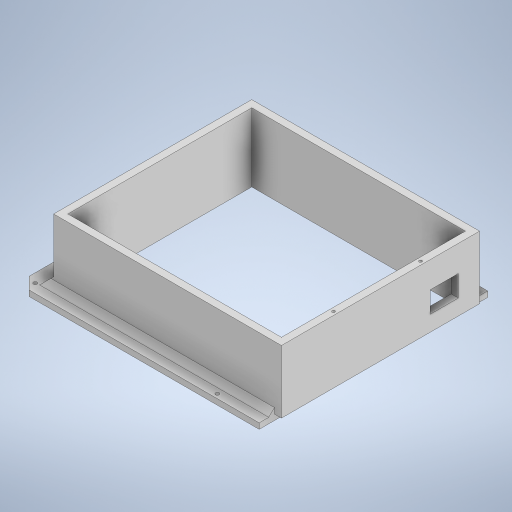
# Autodesk Inventor part: battery holder
Saved by Autodesk Inventor 2023 (Build 270158000, 158)
## iProperties
Created: 2023-08-22
Part Number: battery holder
Material: Generic
Document SubType Name: Modeling
Designer: alian
Density: 1 g/cm^3
Appearance: Default
Author: alian
Autodesk Inventor part; units mm, degrees
ref_plane "YZ Plane" through (0, 0, 0) normal (1, 0, 0) x (0, 1, 0)
ref_plane "XZ Plane" through (0, 0, 0) normal (0, 1, 0) x (-1, 0, 0)
ref_plane "XY Plane" through (0, 0, 0) normal (0, 0, 1) x (1, 0, 0)
sketch "Sketch1" plane through (0, 0, 0) normal (0, 1, 0) x (-1, 0, 0)
  line L0 (0, 0) -> (161, 0)
  line L1 (161, 0) -> (161, -140)
  line L2 (161, -140) -> (0, -140)
  line L3 (0, -140) -> (0, 0)
  line L4 (156, -135) -> (156, -5)
  line L5 (156, -5) -> (5, -5)
  line L6 (5, -5) -> (5, -135)
  line L7 (5, -135) -> (156, -135)
  dimension "d28" = 151
  dimension "d29" = 130
  dimension "d30" = 5
  constraints: 16 end point, 4 parallel, 2 perpendicular, 1 horizontal, 3 other
  measures "d28" distance between parallel lines of L6 L4
  measures "d29" distance between parallel lines of L5 L7
  measures "d30" distance between parallel lines of L7 L2
extrude "Extrusion1" add sketch "Sketch1" along normal blind 44.45
sketch "Sketch2" plane through (0, 0, 0) normal (0, -1, 0) x (1, 0, 0)
  line L0 (-176, 10.75) -> (-5, 10.75)
  line L1 (-5, -150.75) -> (-176, -150.75)
  line L2 (-176, -150.75) -> (-176, 10.75)
  line L3 (-161, 0) -> (0, 0) projected
  line L4 (0, -140) -> (-161, -140) projected
  line L5 (-161, -140) -> (-161, 0) projected
  line L6 (0, -140) -> (-161, -140) projected
  line L7 (0, 0) -> (0, -140) projected
  line L8 (-161, 0) -> (0, 0) projected
  line L9 (-161, -140) -> (-161, 0) projected
  line L10 (-156, -135) -> (-5, -135) projected
  line L11 (-156, -5) -> (-156, -135) projected
  line L12 (-5, -5) -> (-156, -5) projected
  line L13 (-5, -135) -> (-5, -5) projected
  line L14 (-5, 10.75) -> (-5, -5)
  line L15 (-5, -135) -> (-5, -150.75)
  dimension "d31" = 161.5
  dimension "d32" = 171
  constraints: 12 end point, 3 parallel, 2 perpendicular, 1 collinear, 1 horizontal, 1 vertical alignment
  measures "d31" distance between parallel lines of L1 L0
  measures "d32" distance between parallel lines of L15 L2
extrude "Extrusion2" add sketch "Sketch2" along normal blind 4 contours L0 L14 L3 L5 L4 L15 L1 L2 | L14 L12 L11 L10 L15 L4 L5 L3
chamfer "Chamfer1" distance 8.5 angle 45 2 edges at (-176, -2, 10.75) (-176, -2, -150.75)
sketch "Sketch3" plane through (0, 0, 0) normal (0, 1, 0) x (1, 0, 0)
  circle A0 centre (-169.6287, -4.3787) radius 1.25
  circle A1 centre (-37.5, -7.75) radius 1.25
  circle A2 centre (-173, 70) radius 1.25
  circle A3 centre (-169.6287, 144.3787) radius 1.25
  circle A4 centre (-37.5, 147.75) radius 1.25
  line L0 (-176, -10.75) -> (-176, 150.75) projected
  line L1 (-5, -10.75) -> (-176, -10.75) projected
  line L2 (-176, 150.75) -> (-5, 150.75) projected
  line L3 (-161, 123.75) -> (-168, 123.75)
  line L4 (-168, 123.75) -> (-168, 103.75)
  line L5 (-168, 103.75) -> (-161, 103.75)
  line L6 (-161, 103.75) -> (-161, 123.75)
  line L7 (-167.5, -10.75) -> (-176, -2.25) projected
  line L8 (-176, 142.25) -> (-167.5, 150.75) projected
  line L9 (-171.75, -6.5) -> (-169.6287, -4.3787) construction
  line L10 (-171.75, 146.5) -> (-169.6287, 144.3787) construction
  point P0 (0, 0)
  point P1 (-176, 70)
  point P2 (-176, 70)
  point P3 (-164.5, 103.75)
  point P4 (-164.5, 123.75)
  point P5 (-168, 113.75)
  point P6 (-161, 113.75)
  dimension "d10" = 2.5
  dimension "d11" = 2.5
  dimension "d12" = 2.5
  dimension "d13" = 2.5
  dimension "d14" = 2.5
  dimension "d33" = 138.5
  dimension "d35" = 3
  dimension "d37" = 3
  dimension "d38" = 3
  dimension "d58" = 3
  dimension "d59" = 3
  dimension "d60" = 20
  dimension "d61" = 7
  dimension "d62" = 8
  dimension "d63" = 27
  constraints: 12 end point, 8 midpoint, 5 centre point, 4 coincident, 3 perpendicular, 2 parallel, 1 horizontal, 1 horizontal alignment, 1 vertical alignment
  measures "d10" diameter of A0
  measures "d11" diameter of A1
  measures "d12" diameter of A2
  measures "d13" diameter of A3
  measures "d14" diameter of A4
  measures "d33" distance from line of A1.centre L0
  measures "d35" distance from line of L1 A1.centre
  measures "d37" distance from line of L2 A4.centre
  measures "d38" distance from line of L0 A2.centre
  measures "d58" distance of L9.start L9.end
  measures "d59" distance of L10.start L10.end
  measures "d60" distance of point (-164.5, 103.75) point (-164.5, 123.75)
  measures "d61" distance of point (-168, 113.75) point (-161, 113.75)
  measures "d62" distance from line of L0 point (-168, 113.75)
  measures "d63" distance from line of L2 point (-164.5, 123.75)
extrude "Extrusion3" cut sketch "Sketch3" against normal blind 11.1125 contours A0 | A1 | A2 | A3 | A4 | L6 L5 L4 L3
sketch "Sketch4" plane through (0, 44.45, 0) normal (0, 1, 0) x (1, 0, 0)
  circle A0 centre (-2.5, 100.75) radius 1
  circle A1 centre (-2.5, 39.25) radius 1
  line L0 (-161, 0) -> (0, 0) projected
  line L1 (0, 140) -> (-161, 140) projected
  line L2 (0, 140) -> (-5, 140) projected
  line L3 (-167.5, 150.75) -> (-5, 150.75) projected
  line L4 (-5, -10.75) -> (-167.5, -10.75) projected
  point P0 (-2.5, 140)
  dimension "d20" = 2
  dimension "d39" = 50
  dimension "d51" = 50
  constraints: 2 centre point, 2 vertical alignment, 1 equal radius, 1 midpoint
  measures "d20" diameter of A1
  measures "d39" distance from line of L3 A0.centre
  measures "d51" distance from line of A1.centre L4
extrude "Extrusion4" cut sketch "Sketch4" against normal blind 65.0875
chamfer "Chamfer2" distance 4 angle 45 2 edges at (-83, 0, 0) (-83, 0, -140)
chamfer "Chamfer3" distance 6 angle 45 2 edges at (-161, 0, -51.875) (-161, 0, -131.875)
sketch "Sketch6" plane through (0, 0, 0) normal (1, 0, 0) x (0, 0, -1)
  line L0 (105, 26) -> (125, 26)
  line L1 (125, 26) -> (125, 11)
  line L2 (125, 11) -> (105, 11)
  line L3 (105, 11) -> (105, 26)
  line L4 (5, -4) -> (-10.75, -4) projected
  line L5 (0, 0) -> (0, 44.45) projected
  line L6 (140, 0) -> (140, 44.45) projected
  point P0 (125, 18.5)
  point P1 (105, 18.5)
  dimension "d64" = 15
  dimension "d65" = 15
  dimension "d66" = 20
  dimension "d70" = 15
  constraints: 8 end point, 2 midpoint, 2 parallel, 1 horizontal, 1 perpendicular
  measures "d64" distance between parallel lines of L4 L2
  measures "d65" distance between parallel lines of L0 L2
  measures "d66" distance of point (125, 18.5) point (105, 18.5)
  measures "d70" distance between parallel lines of L1 L6
extrude "Extrusion6" cut sketch "Sketch6" against normal blind 9.05
equation "\"d11\" = d10"
equation "\"d12\" = d11"
equation "\"d13\" = d12"
equation "\"d14\" = d12"
equation "\"d35\" = d34"
equation "\"d37\" = d36"
equation "\"d38\" = d34"
equation "\"d36\" = d34"
equation "\"d34\" = 3"
body "Solid1"
